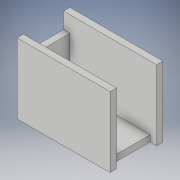
# Autodesk Inventor part: Base_servo1
Saved by Autodesk Inventor 2019 (Build 230136000, 136)
## iProperties
Created: 2020-02-05
Part Number: Base_servo1
Material: Generic
Document SubType Name: Modeling
Designer: Omar
Density: 1 g/cm^3
Appearance: Default
Author: Omar
Autodesk Inventor part; units mm, degrees
ref_plane "YZ Plane" through (0, 0, 0) normal (1, 0, 0) x (0, 1, 0)
ref_plane "XZ Plane" through (0, 0, 0) normal (0, 1, 0) x (-1, 0, 0)
ref_plane "XY Plane" through (0, 0, 0) normal (0, 0, 1) x (1, 0, 0)
sketch "Sketch2" plane through (0, 0, 0) normal (0, 1, 0) x (-1, 0, 0)
  line L0 (0, 0) -> (40, 0)
  line L1 (40, 0) -> (40, -20)
  line L2 (40, -20) -> (0, -20)
  line L3 (0, -20) -> (0, 0)
  dimension "d25" = 40
  dimension "d26" = 20
  constraints: 8 end point, 2 parallel, 1 horizontal, 1 perpendicular
  measures "d25" distance of L1.end L2.end
  measures "d26" distance of L0.end L1.end
extrude "Extrusion1" add sketch "Sketch2" along normal blind 3.18
sketch "Sketch5" plane through (0, 0, 0) normal (0, 1, 0) x (-1, 0, 0)
  line L0 (40, 0) -> (0, 0) projected
  line L1 (0, 0) -> (0, -20) projected
  line L2 (0, -20) -> (40, -20) projected
  line L3 (40, -20) -> (40, 0) projected
  line L4 (-3.18, 0) -> (43.18, 0)
  line L5 (43.18, 0) -> (43.18, 3.18)
  line L6 (43.18, 3.18) -> (-3.18, 3.18)
  line L7 (-3.18, 3.18) -> (-3.18, 0)
  line L8 (43.18, -20) -> (-3.18, -20)
  line L9 (-3.18, -20) -> (-3.18, -23.18)
  line L10 (-3.18, -23.18) -> (43.18, -23.18)
  line L11 (43.18, -23.18) -> (43.18, -20)
  dimension "d34" = 3.18
  dimension "d35" = 3.18
  dimension "d36" = 3.18
  constraints: 16 end point, 4 collinear, 4 parallel, 2 horizontal, 2 perpendicular, 1 point on line
  measures "d34" distance between parallel lines of L5 L3
  measures "d35" distance between parallel lines of L1 L7
  measures "d36" distance between parallel lines of L4 L6
extrude "Extrusion2" add sketch "Sketch5" along normal blind 35 contours L0 L4 L7 L6 L5 | L8 L11 L10 L9 L2
sketch "Sketch6" plane through (0, 0, 0) normal (0, 1, 0) x (-1, 0, 0)
  line L0 (40, 0) -> (0, 0) projected
  line L1 (0, 0) -> (0, -20) projected
  line L2 (0, -20) -> (40, -20) projected
  line L3 (40, -20) -> (40, 0) projected
  line L4 (40, 0) -> (43.18, 0)
  line L5 (43.18, 0) -> (43.18, -20)
  line L6 (43.18, -20) -> (40, -20)
  line L7 (40, -20) -> (40, 0)
  dimension "d39" = 3.18
  dimension "d40" = 20
  constraints: 8 end point, 2 parallel, 1 horizontal, 1 perpendicular
  measures "d39" distance of L5.end L6.end
  measures "d40" distance of L4.end L5.end
extrude "Extrusion3" add sketch "Sketch6" along normal blind 27 contours L4 L5 L6 L3
body "Solid1"
